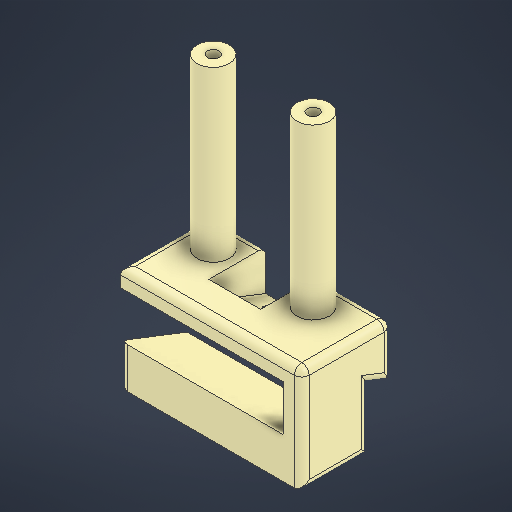
# Autodesk Inventor part: astra_holder
Saved by Autodesk Inventor 2026 (Build 300175050, 175E)
## iProperties
Created: 2025-06-12
Part Number: astra_holder
Material: Generic
Document SubType Name: Modeling
Designer: satom
Density: 1 g/cm^3
Appearance: Default
Author: satom
Autodesk Inventor part; units mm, degrees
ref_plane "YZ Plane" through (0, 0, 0) normal (1, 0, 0) x (0, 1, 0)
ref_plane "XZ Plane" through (0, 0, 0) normal (0, 1, 0) x (-1, 0, 0)
ref_plane "XY Plane" through (0, 0, 0) normal (0, 0, 1) x (1, 0, 0)
sketch "Sketch1" plane through (0, 0, 0) normal (1, 0, 0) x (0, 1, 0)
  line L0 (0, 0) -> (0, -22.86)
  line L1 (0, -22.86) -> (5.08, -22.86)
  line L2 (5.08, -22.86) -> (13.97, 0)
  line L3 (13.97, 0) -> (0, 0)
  dimension "d0" = 22.86
  dimension "d1" = 5.08
  dimension "d2" = 13.97
  constraints: 8 end point, 1 parallel, 1 perpendicular, 1 vertical
  measures "d0" distance of L0.start L0.end
  measures "d1" distance of L0.end L1.end
  measures "d2" distance of L2.end L0.start
extrude "Extrusion1" add sketch "Sketch1" along normal blind 55.88
sketch "Sketch2" plane through (55.88, 0, 0) normal (1, 0, 0) x (0, 0, -1)
  line L0 (0, 0) -> (22.9656, 0)
  line L1 (22.9656, 0) -> (22.9656, 29.6925)
  line L2 (22.9656, 29.6925) -> (0, 29.6925)
  line L3 (0, 29.6925) -> (0, 0)
  dimension "d5" = 29.6925
  constraints: 8 end point, 2 parallel, 1 horizontal, 1 perpendicular
  measures "d5" distance of L0.end L1.end
extrude "Extrusion2" add sketch "Sketch2" along normal blind 6.35
sketch "Sketch3" plane through (55.88, 0, 0) normal (-1, 0, 0) x (0, 0, 1)
  line L0 (-22.9656, 29.6925) -> (0, 29.6925) projected
  line L1 (0, 29.6925) -> (-30.7748, 29.6925)
  line L2 (-30.7748, 29.6925) -> (-30.7748, 17.7245)
  line L3 (-30.7748, 17.7245) -> (0, 29.6925)
  point P0 (0, 0)
  dimension "d8" = 33.02
  dimension "d9" = 11.968
  constraints: 6 end point, 1 horizontal, 1 perpendicular
  measures "d8" distance of L2.end L0.end
  measures "d9" distance of L1.end L2.end
extrude "Extrusion3" add sketch "Sketch3" along normal blind 55.88
sketch "Sketch4" plane through (0, 0, 0) normal (-1, 0, 0) x (0, 0, 1)
  line L0 (-30.7748, 29.6925) -> (-30.7748, 17.7245) projected
  line L1 (-30.7748, 22.1078) -> (-11.2714, 29.6925)
  line L2 (-22.9656, 29.6925) -> (0, 29.6925) projected
  line L3 (-30.7748, 17.7245) -> (0, 29.6925) projected
  line L4 (-30.7748, 22.1078) -> (-30.7748, 29.6925)
  line L5 (0, 29.6925) -> (-30.7748, 29.6925) projected
  point P0 (0, 0)
  dimension "d12" = 4.0853
  dimension "d13" = 7.5846
  dimension "d14" = 19.5034
  constraints: 4 end point, 2 point on line, 1 collinear, 1 parallel
  measures "d12" distance between parallel lines of L1 L3
  measures "d13" distance from line of L5 L1.start
  measures "d14" distance of L1.end L0.start
extrude "Extrusion4" cut sketch "Sketch4" against normal blind 55.88 contours L5 L2 L1 L0
sketch "Sketch5" plane through (0, 0, 0) normal (-1, 0, 0) x (0, 0, 1)
  line L0 (-22.9656, 29.6925) -> (0, 29.6925) projected
  line L1 (-30.7748, 22.1078) -> (-30.7748, 17.7245) projected
  line L2 (-11.2714, 29.6925) -> (-30.7748, 22.1078)
  line L3 (-30.7748, 22.1078) -> (-30.7748, 29.6925)
  line L4 (-30.7748, 29.6925) -> (-11.1381, 29.6925)
  line L5 (-11.2714, 29.6925) -> (-30.7748, 22.1078) projected
  point P0 (0, 0)
  constraints: 6 end point, 2 collinear, 2 point on line, 1 perpendicular
extrude "Extrusion5" add sketch "Sketch5" against normal blind 19.05
sketch "Sketch6" plane through (55.88, 0, 0) normal (1, 0, 0) x (0, 0, -1)
  line L0 (30.7748, 22.1078) -> (30.7748, 29.6925) projected
  line L1 (30.7748, 29.6925) -> (30.7748, 22.1078)
  line L2 (30.7748, 22.1078) -> (11.2714, 29.6925) projected
  line L3 (30.7748, 22.1078) -> (11.2714, 29.6925)
  line L4 (11.2714, 29.6925) -> (30.7748, 29.6925)
  point P0 (0, 0)
  point P1 (11.4828, 29.6925)
  constraints: 6 end point, 1 collinear, 1 perpendicular, 1 vertical
extrude "Extrusion6" add sketch "Sketch6" against normal blind 19.05
sketch "Sketch7" plane through (0, 29.6925, -11.2714) normal (0, 0.9320047, -0.3624463) x (1, 0, 0)
  line L0 (36.83, 0) -> (19.05, 0) construction
  circle A0 centre (27.94, 14.2202) radius 2.8575
  line L1 (19.05, 20.9262) -> (36.83, 20.9262) projected
  line L2 (19.05, 18.1772) -> (19.05, 0) projected
  point P0 (0, 0.2569)
  point P1 (27.94, 0)
  point P2 (0, 0)
  point P3 (0, 20.9262)
  point P4 (55.88, 20.9262)
  dimension "d21" = 5.715
  dimension "d39" = 6.7061
  dimension "d40" = 8.89
  constraints: 1 centre point, 1 midpoint
  measures "d21" diameter of A0
  measures "d39" distance from line of L1 A0.centre
  measures "d40" distance from line of L2 A0.centre
extrude "Extrusion7" cut sketch "Sketch7" against normal up to next
sketch "Sketch8" plane through (62.23, 29.6925, 0) normal (0, 1, 0) x (1, 0, 0)
  line L0 (-6.35, 22.9656) -> (0, 22.9656) construction
  circle A0 centre (-17.145, 21.0231) radius 5.5563
  circle A1 centre (-51.435, 21.0231) radius 5.5563
  line L1 (-25.4, 11.2714) -> (-25.4, 30.7748) construction
  line L2 (-25.4, 21.0231) -> (0, 21.0231) construction
  line L3 (0, 22.9656) -> (0, 0) construction
  line L4 (-43.18, 30.7748) -> (-43.18, 11.2714) construction
  line L5 (-43.18, 21.0231) -> (-59.69, 21.0231) construction
  line L6 (-25.4, 11.2714) -> (-43.18, 11.2714) construction
  line L7 (-34.29, 11.2714) -> (-34.29, 30.7748) construction
  line L8 (-6.35, 30.7748) -> (-62.23, 30.7748) construction
  point P0 (-62.23, 0)
  point P1 (-62.23, 11.2714)
  point P2 (-51.435, 21.0231)
  dimension "d26" = 11.1125
  dimension "d27" = 11.1125
  dimension "d43" = 17.145
  dimension "d46" = 17.145
  constraints: 6 end point, 6 midpoint, 3 point on line, 2 centre point, 1 horizontal
  measures "d26" diameter of A0
  measures "d27" diameter of A1
  measures "d43" distance from line of A0.centre L7
  measures "d46" distance from line of L7 A1.centre
extrude "Extrusion8" add sketch "Sketch8" along normal blind 64.262
sketch "Sketch9" plane through (45.085, 93.9545, -21.0231) normal (0, 1, 0) x (1, 0, 0)
  circle A0 centre (0, 0) radius 5.5562 construction
  line L0 (0, -5.5562) -> (0, 5.5562) construction
  line L1 (5.7118, 0) -> (-5.6102, 0) construction
  circle A1 centre (-34.29, 0) radius 5.5562 construction
  line L2 (-28.7338, 0) -> (-39.8463, 0) construction
  line L3 (-34.29, 5.5562) -> (-34.29, -5.5562) construction
  circle A2 centre (0, 0) radius 2
  circle A3 centre (-34.29, 0) radius 2
  point P0 (-45.085, -21.0231)
  dimension "d47" = 4
  dimension "d48" = 4
  constraints: 8 end point, 6 point on circle, 2 centre point, 2 coincident, 2 point on line, 1 horizontal, 1 perpendicular, 1 vertical
  measures "d47" diameter of A2
  measures "d48" diameter of A3
extrude "Extrusion9" cut sketch "Sketch9" against normal blind 7
sketch "Sketch10" plane through (55.88, 0, 0) normal (1, 0, 0) x (0, 0, -1)
  line L0 (22.9656, 0) -> (22.9656, 29.6925) projected
  line L1 (30.7748, 29.6925) -> (22.9656, 29.6925)
  line L2 (25.7072, 19.6952) -> (20.3808, 21.7666) projected
  line L3 (30.7748, 17.7245) -> (30.7748, 29.6925)
  line L4 (22.9656, 29.6925) -> (22.9656, 20.7614)
  line L5 (22.9656, 20.7614) -> (30.7748, 17.7245)
  point P0 (0, 0)
  constraints: 8 end point, 1 perpendicular, 1 point on line
extrude "Extrusion10" add sketch "Sketch10" along normal up to surface (6.35 mm away)
sketch "Sketch11" plane through (0, 29.6925, 0) normal (0, 1, 0) x (1, 0, 0)
  line L0 (62.23, 0) -> (62.23, 30.7748) projected
  line L1 (62.23, 0) -> (0, 0)
  line L2 (62.23, 30.7748) -> (0, 30.7748) projected
  line L3 (0, 0) -> (0, 30.7748)
  line L4 (19.05, 30.7748) -> (19.05, 11.2714) projected
  line L5 (0, 30.7748) -> (19.05, 30.7748)
  line L6 (19.05, 30.7748) -> (19.05, 11.2714)
  line L7 (36.83, 11.2714) -> (36.83, 30.7748) projected
  line L8 (19.05, 11.2714) -> (36.83, 11.2714)
  line L9 (36.83, 11.2714) -> (36.83, 30.7748)
  line L10 (36.83, 30.7748) -> (62.23, 30.7748)
  line L11 (62.23, 30.7748) -> (62.23, 0)
  line L12 (0, 0) -> (62.23, 0)
  constraints: 18 end point, 5 perpendicular, 2 collinear, 1 horizontal, 1 point on line
extrude "Extrusion11" add sketch "Sketch11" along normal blind 6.35 contours L1 L3 L2 L4 L8 L7 L0
fillet "Fillet1" radius 2.54 12 edges at (49.53, 36.0425, -30.7748) (9.525, 36.0425, -30.7748) (62.23, 36.0425, -15.3874) (31.115, 36.0425, 0) (0, 36.0425, -15.3874) (62.23, 18.0212, 0) (62.23, 0, -11.4828) (62.23, 10.3807, -22.9656) (62.23, 19.243, -26.8702) (62.23, 26.8835, -30.7748) (0, 26.8835, -30.7748) (0, 6.985, 0)
equation "\"d46\" = d43"
equation "\"d47\" = m3_heat_set_insert"
equation "\"d48\" = m3_heat_set_insert"
equation "\"d35\" = m3_heat_set_depth"
equation "\"m3_heat_set_insert\" = 4"
equation "\"m3_clearance\" = 3.4"
equation "\"m3_heat_set_depth\" = 7"
equation "\"robot_diameter\" = 354"
equation "\"hardboard_thickness\" = 5"
equation "\"motor_centerline_height\" = 13"
body "Solid1"
